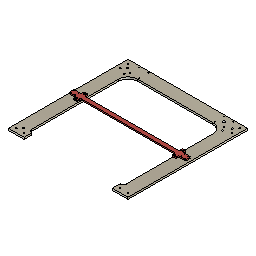
mark 4 top plate nema 23 version (Autodesk Fusion 360 design; units mm, degrees)
Autodesk Fusion 360 part; units mm, degrees
sketch "Sketch1" plane through (0, 0, 0) normal (0, 0, 1) x (1, 0, 0)
  circle A0 centre (2220.6568, 497.0935) radius 8 construction
  circle A1 centre (2186.2292, 516.3803) radius 8 construction
  circle A2 centre (2186.2292, 539.9503) radius 6.25
  line L0 (2209.7992, 516.3803) -> (2162.6592, 516.3803) construction
  circle A3 centre (2209.7992, 516.3803) radius 2.5
  line L1 (2209.7992, 563.5203) -> (2209.7992, 516.3803) construction
  line L2 (2180.9147, 536.6612) -> (2192.6086, 521.2077) construction
  circle A4 centre (2162.6592, 563.5203) radius 2.5
  line L3 (2162.6592, 516.3803) -> (2162.6592, 563.5203) construction
  line L4 (2162.6592, 563.5203) -> (2209.7992, 563.5203) construction
  circle A5 centre (1718.6797, 497.092) radius 8 construction
  circle A6 centre (1753.2073, 516.3788) radius 8 construction
  circle A7 centre (1753.2073, 539.9488) radius 6.25 construction
  line L5 (1729.6373, 516.3788) -> (1776.7773, 563.5188) construction
  line L6 (1729.6373, 516.3788) -> (1776.7773, 516.3788) construction
  circle A8 centre (1729.6373, 516.3788) radius 2.5
  line L7 (1729.6373, 563.5188) -> (1729.6373, 516.3788) construction
  circle A9 centre (1776.7773, 563.5188) radius 2.5
  line L8 (1776.7773, 516.3788) -> (1776.7773, 563.5188) construction
  line L9 (1776.7773, 563.5188) -> (1729.6373, 563.5188) construction
  circle A10 centre (1776.7773, 516.3788) radius 2.5006
  circle A11 centre (1729.6373, 563.5188) radius 2.5006
  circle A12 centre (2209.7992, 563.5203) radius 2.5
  circle A13 centre (2162.6592, 516.3803) radius 2.5
  circle A14 centre (2236.6726, 530.4061) radius 4
  circle A15 centre (1702.7758, 530.4098) radius 4
  circle A16 centre (1718.6797, 497.092) radius 4
  circle A17 centre (2220.6568, 497.0935) radius 4
  circle A18 centre (2236.6726, 530.4061) radius 8 construction
  circle A19 centre (1702.7758, 530.4098) radius 8 construction
  circle A20 centre (2254.5183, 550.8989) radius 3.5
  circle A21 centre (2254.5183, 510.8989) radius 3.5
  circle A22 centre (1685, 550.8955) radius 3.5
  line L10 (1685, 550.8955) -> (1685, 510.8955) construction
  circle A23 centre (1685, 510.8955) radius 3.5
  line L11 (1744.9182, -38.7028) -> (1744.9182, 1.2972)
  line L12 (1744.9182, 1.2972) -> (1743.5, 1.2972)
  line L13 (2194.5182, -38.7028) -> (2194.5182, 1.2972)
  line L14 (2194.5182, 1.2972) -> (2196.0182, 1.2972)
  line L15 (1778.5, 507.7284) -> (2161.0182, 507.7284)
  line L16 (2274.5182, -38.7028) -> (2194.5182, -38.7028)
  line L17 (1744.9182, -38.7028) -> (1664.9182, -38.7028)
  arc A24 (1778.5, 507.7284) -> (1728.5, 457.7284) centre (1778.5, 457.7284) ccw
  arc A25 (2211.0182, 457.7284) -> (2161.0182, 507.7284) centre (2161.0182, 457.7284) ccw
  arc A26 (1728.5, 16.2972) -> (1743.5, 1.2972) centre (1743.5, 16.2972) ccw
  arc A27 (2196.0182, 1.2972) -> (2211.0182, 16.2972) centre (2196.0182, 16.2972) ccw
  circle A28 centre (1684.9182, -18.7028) radius 3.5
  circle A29 centre (1724.9182, -18.7028) radius 3.5
  circle A30 centre (2214.5182, -18.7028) radius 3.5
  circle A31 centre (2254.5182, -18.7028) radius 3.5
  line L18 (2274.5182, -38.7028) -> (2274.5182, 570.8972)
  line L19 (2274.5182, 570.8972) -> (1665, 570.8955)
  line L20 (1665, 570.8955) -> (1664.9182, -38.7028)
  circle A32 centre (2236.6726, 0.4061) radius 8 construction
  line L21 (1672.1777, 267) -> (1672.1777, 284)
  line L22 (2267.1777, 284) -> (2267.1777, 267)
  line L23 (1708.8553, 292) -> (1708.8553, 299)
  line L24 (1712.8553, 303) -> (1724.5, 303)
  line L25 (1728.5, 299) -> (1728.5, 292)
  line L26 (1724.5, 248) -> (1712.8553, 248)
  line L27 (1708.8553, 252) -> (1708.8553, 259)
  line L28 (1728.5, 259) -> (1728.5, 252)
  line L29 (2226.5, 248) -> (2215.0182, 248)
  line L30 (2210.8553, 256.2827) -> (2210.8553, 259)
  line L31 (2210.8553, 263) -> (2211.0182, 263)
  line L32 (2230.5, 259) -> (2230.5, 252)
  line L33 (2210.8553, 248) -> (2211.0182, 248.1244) construction
  line L34 (2211.0182, 288) -> (2210.8553, 288)
  line L35 (2210.8553, 292) -> (2210.8553, 299)
  line L36 (2214.8553, 303) -> (2226.5, 303)
  line L37 (2230.5, 299) -> (2230.5, 292)
  line L38 (2263.1777, 263) -> (2234.5, 263)
  line L39 (2234.5, 288) -> (2263.1777, 288)
  line L40 (2211.0182, 262.8756) -> (2210.8553, 263) construction
  line L41 (1704.8553, 263) -> (1676.1777, 263)
  line L42 (1728.5, 457.7284) -> (1728.5, 292)
  line L43 (1728.5, 259) -> (1728.5, 16.2972)
  line L44 (1676.1777, 288) -> (1704.8553, 288)
  arc A33 (1708.8553, 259) -> (1704.8553, 263) centre (1704.8553, 259) ccw
  arc A34 (1704.8553, 288) -> (1708.8553, 292) centre (1704.8553, 292) ccw
  arc A35 (2230.5, 292) -> (2234.5, 288) centre (2234.5, 292) ccw
  arc A36 (2234.5, 263) -> (2230.5, 259) centre (2234.5, 259) ccw
  arc A37 (2226.5, 248) -> (2230.5, 252) centre (2226.5, 252) ccw
  arc A38 (2211.0182, 252) -> (2215.0182, 248) centre (2215.0182, 252) ccw
  arc A39 (2214.8553, 303) -> (2210.8553, 299) centre (2214.8553, 299) ccw
  arc A40 (2230.5, 299) -> (2226.5, 303) centre (2226.5, 299) ccw
  arc A41 (2263.1777, 263) -> (2267.1777, 267) centre (2263.1777, 267) ccw
  arc A42 (2267.1777, 284) -> (2263.1777, 288) centre (2263.1777, 284) ccw
  arc A43 (1672.1777, 267) -> (1676.1777, 263) centre (1676.1777, 267) ccw
  arc A44 (1676.1777, 288) -> (1672.1777, 284) centre (1676.1777, 284) ccw
  arc A45 (1712.8553, 303) -> (1708.8553, 299) centre (1712.8553, 299) ccw
  arc A46 (1728.5, 299) -> (1724.5, 303) centre (1724.5, 299) ccw
  arc A47 (1724.5, 248) -> (1728.5, 252) centre (1724.5, 252) ccw
  arc A48 (1708.8553, 252) -> (1712.8553, 248) centre (1712.8553, 252) ccw
  line L45 (2211.0182, 262.8756) -> (2211.0182, 263)
  line L46 (2211.0182, 288) -> (2211.0182, 288.1244)
  line L47 (2211.0182, 252) -> (2210.8553, 256.2827)
  circle A49 centre (1718.6777, 295.5) radius 4
  circle A50 centre (1718.6777, 255.5) radius 4
  circle A51 centre (2220.6777, 295.5) radius 4
  circle A52 centre (2220.3553, 255.5) radius 4
  circle A53 centre (2240.6777, 283) radius 1.5
  circle A54 centre (2240.6777, 268) radius 1.5
  circle A55 centre (2260.6777, 268) radius 1.5
  circle A56 centre (2260.6777, 283) radius 1.5
  circle A57 centre (1698.6777, 283) radius 1.5
  circle A58 centre (1698.6777, 268) radius 1.5
  circle A59 centre (1678.6777, 268) radius 1.5
  circle A60 centre (1678.6777, 283) radius 1.5
  circle A61 centre (1718.6777, 255.5) radius 8 construction
  circle A62 centre (1718.6777, 295.5) radius 8 construction
  circle A63 centre (2220.3553, 255.5) radius 8 construction
  circle A64 centre (2220.6777, 295.5) radius 8 construction
  line L48 (2228.3553, 255.5) -> (2228.3553, 0.4062) construction
  line L49 (2244.6726, 0.4059) -> (2244.6726, 530.4061) construction
  line L50 (1664.9159, -55.9986) -> (1702.7616, -56.0037)
  circle A65 centre (1702.7692, 0.4768) radius 4
  circle A66 centre (1702.7692, 0.4768) radius 8 construction
  line L51 (1694.7692, 0.4768) -> (1694.7692, 530.8955) construction
  line L52 (1710.7692, 0.4768) -> (1710.6777, 255.4971) construction
  line L53 (2205.8553, 265.5) -> (1733.5, 265.5)
  line L54 (1733.5, 285.5) -> (2205.8553, 285.5)
  line L55 (1728.5, 292) -> (1728.5, 290.5)
  line L56 (1728.5, 259) -> (1728.5, 260.5)
  line L57 (2210.8553, 292) -> (2210.8553, 290.5)
  line L58 (2210.8553, 259) -> (2210.8553, 260.5)
  arc A67 (1728.5, 290.5) -> (1733.5, 285.5) centre (1733.5, 290.5) ccw
  arc A68 (1733.5, 265.5) -> (1728.5, 260.5) centre (1733.5, 260.5) ccw
  arc A69 (2205.8553, 285.5) -> (2210.8553, 290.5) centre (2205.8553, 290.5) ccw
  arc A70 (2210.8553, 260.5) -> (2205.8553, 265.5) centre (2205.8553, 260.5) ccw
  line L59 (2187.667, 546.0327) -> (2237.888, 538.3132) construction
  line L60 (1710.6777, 295.5) -> (1710.6777, 497.092) construction
  line L61 (2228.6777, 295.5) -> (2228.6777, 497.0935) construction
  line L62 (1748, 523) -> (1758.1512, 536.1251)
  line L63 (1751.7695, 546.0312) -> (1701.5609, 538.317)
  line L64 (1753.2073, 508.3788) -> (2220.6568, 505.0935) construction
  line L65 (2186.2292, 508.3803) -> (1718.6234, 505.0918) construction
  line L66 (1999.6777, 245.5) -> (1939.6777, 245.5) construction
  line L67 (1939.6777, 245.5) -> (1939.6777, 305.5) construction
  line L68 (1939.6777, 305.5) -> (1999.6777, 305.5) construction
  line L69 (1999.6777, 305.5) -> (1999.6777, 245.5) construction
  line L70 (1999.6777, 245.5) -> (1939.6777, 305.5) construction
  line L71 (1939.6777, 245.5) -> (1999.6777, 305.5) construction
  line L72 (2220.6777, 287.5) -> (1999.6777, 287.5) construction
  line L73 (2220.3553, 263.5) -> (1999.6777, 263.5) construction
  line L74 (1718.6777, 263.5) -> (1939.6777, 263.5) construction
  line L75 (1718.6777, 287.5) -> (1939.6777, 287.5) construction
  line L76 (2211.0182, 457.7284) -> (2211.0182, 16.2972)
  line L77 (1728.5, 241.8932) -> (1728.5, 309)
  point P0 (2186.2292, 539.9503)
  point P1 (2220.6568, 505.0935)
  point P2 (2186.2292, 516.3803)
  point P3 (2220.6568, 497.0935)
  point P4 (2186.2292, 516.3803)
  point P5 (2186.2292, 539.9503)
  point P6 (2220.6568, 497.0935)
  point P7 (2186.2292, 539.9503)
  point P8 (2187.667, 546.0327)
  point P9 (2186.2292, 508.3803)
  point P10 (1753.2073, 539.9488)
  point P11 (1722.3963, 504.1763)
  point P12 (1753.2073, 516.3788)
  point P13 (1718.6797, 497.092)
  point P14 (1753.2073, 516.3788)
  point P15 (1753.2073, 539.9488)
  point P16 (1718.6797, 497.092)
  point P17 (1753.2073, 539.9488)
  point P18 (1751.7695, 546.0312)
  point P19 (1753.2073, 508.3788)
  point P20 (2236.6726, 530.4061)
  point P21 (1702.7758, 530.4098)
  point P22 (1724.9182, -18.7028)
  point P23 (1684.9182, -18.7028)
  point P24 (2214.5182, -18.7028)
  point P25 (2254.5182, -18.7028)
  point P26 (1665, 570.8955)
  point P27 (2274.5182, 570.8972)
  point P28 (2236.6726, 0.4061)
  point P29 (1969.6777, 275.5)
  point P30 (1718.6777, 295.5)
  point P31 (1718.6777, 255.5)
  point P32 (2220.6777, 295.5)
  point P33 (2220.3553, 255.5)
  point P34 (1698.6777, 283)
  point P35 (1698.6777, 268)
  point P36 (1678.6777, 283)
  point P37 (1678.6777, 268)
  point P38 (2260.6777, 283)
  point P39 (2260.6777, 268)
  point P40 (2240.6777, 268)
  point P41 (2240.6777, 283)
  point P42 (1672.1777, 288)
  point P43 (2267.1777, 288)
  point P44 (1969.6777, 275.5)
  point P45 (1718.6777, 295.5)
  point P46 (1718.6777, 255.5)
  point P47 (2220.6777, 255.5)
  point P48 (2220.6777, 295.5)
  point P49 (1702.7692, 0.4768)
  point P50 (1969.6777, 275.5)
  point P51 (1969.6777, 275.5)
  dimension "d314" = 47.14
  dimension "d315" = 47.14
  dimension "d316" = 5
  dimension "d317" = 5
  dimension "d318" = 12.5
  dimension "d319" = 16
  dimension "d320" = 16
  dimension "d321" = 47.14
  dimension "d322" = 47.14
  dimension "d323" = 5
  dimension "d324" = 5
  dimension "d325" = 12.5
  dimension "d326" = 16
  dimension "d327" = 16
  dimension "d328" = 5.0013
  dimension "d329" = 5.0013
  dimension "d330" = 5
  dimension "d331" = 5
  dimension "d336" = 8
  dimension "d337" = 8
  dimension "d338" = 8
  dimension "d339" = 8
  dimension "d340" = 16
  dimension "d341" = 16
  dimension "d344" = 7
  dimension "d345" = 40
  dimension "d346" = 7
  dimension "d349" = 7
  dimension "d350" = 40
  dimension "d351" = 7
  dimension "d355" = 80
  dimension "d357" = 80
  dimension "d360" = 50
  dimension "d361" = 50
  dimension "d362" = 15
  dimension "d363" = 15
  dimension "d366" = 40
  dimension "d367" = 7
  dimension "d368" = 7
  dimension "d371" = 40
  dimension "d372" = 7
  dimension "d373" = 7
  dimension "d376" = 530
  dimension "d377" = 16
  dimension "d393" = 502
  dimension "d394" = 40
  dimension "d399" = 20
  dimension "d400" = 20
  dimension "d401" = 595
  dimension "d403" = 8
  dimension "d404" = 8
  dimension "d405" = 8
  dimension "d406" = 8
  dimension "d407" = 3
  dimension "d408" = 3
  dimension "d409" = 3
  dimension "d410" = 3
  dimension "d412" = 3
  dimension "d413" = 3
  dimension "d414" = 3
  dimension "d415" = 3
  dimension "d418" = 16
  dimension "d419" = 16
  dimension "d420" = 16
  dimension "d421" = 16
  dimension "d423" = 37.8457
  dimension "d424" = 8
  dimension "d425" = 16
  dimension "d427" = 5
  dimension "d428" = 5
  dimension "d429" = 5
  dimension "d430" = 5
  dimension "d431" = 60
  dimension "d432" = 60
  constraint horizontal L16
  constraint coincident P7 P5
  constraint perpendicular L0 L3
  constraint parallel L0 L4
  constraint parallel L1 L3
  constraint horizontal L0
  constraint coincident A4.centre L3.end
  constraint coincident L0.start A3.centre
  constraint midpoint P4 L0
  constraint coincident P4 P2
  constraint coincident P6 P3
  constraint coincident P8 A2
  constraint coincident L2.start A2
  constraint coincident L2.end A1
  constraint tangent A1 L2
  constraint coincident P9 A1
  constraint coincident P1 A0
  constraint coincident P17 P15
  constraint perpendicular L6 L8
  constraint parallel L6 L9
  constraint parallel L7 L8
  constraint coincident P17 L5
  constraint coincident L5.end A9.centre
  constraint coincident L5.start L6.start
  constraint midpoint P14 L6
  constraint coincident P14 P12
  constraint coincident P16 P13
  constraint coincident P18 A7
  constraint coincident P19 A6
  constraint coincident P11 A5
  constraint coincident L6.end L8.start
  constraint coincident L7.start L9.end
  constraint coincident L1.start L4.end
  constraint coincident L0.end L3.start
  constraint coincident P20 A14.centre
  constraint coincident P21 A15.centre
  constraint concentric A0 A17
  constraint coincident A22.centre L10.start
  constraint coincident L10.end A23.centre
  constraint perpendicular L16 L42
  constraint vertical L11
  constraint horizontal L12
  constraint vertical L13
  constraint horizontal L14
  constraint collinear L16 L17
  constraint tangent A24 L42
  constraint tangent L15 A24
  constraint tangent L15 A25
  constraint tangent L12 A26
  constraint tangent A26 L42
  constraint tangent L14 A27
  constraint coincident P23 A28.centre
  constraint coincident P22 A29.centre
  constraint coincident P24 A30.centre
  constraint coincident P25 A31.centre
  constraint coincident P27 L18.end
  constraint perpendicular L16 L18
  constraint coincident P26 L19.end
  constraint coincident P28 A32.centre
  constraint coincident A32 L49.start
  constraint perpendicular L21 L38
  constraint parallel L38 L44
  constraint parallel L21 L22
  constraint horizontal L38
  constraint parallel L23 L25
  constraint coincident P45 P30
  constraint perpendicular L26 L27
  constraint parallel L27 L28
  constraint horizontal L26
  constraint perpendicular L29 L30
  constraint parallel L29 L31
  constraint parallel L30 L32
  constraint horizontal L29
  constraint coincident L33 P47
  constraint perpendicular L34 L35
  constraint parallel L34 L36
  constraint parallel L35 L37
  constraint horizontal L34
  constraint coincident P48 P32
  constraint collinear L39 L44
  constraint collinear L42 L43
  constraint tangent L27 A33
  constraint tangent L41 A33
  constraint tangent L44 A34
  constraint tangent L23 A34
  constraint coincident L31.start L30
  constraint coincident L34.end L35
  constraint tangent L37 A35
  constraint tangent L39 A35
  constraint tangent L38 A36
  constraint tangent L32 A36
  constraint tangent L29 A37
  constraint tangent L32 A37
  constraint coincident L33.start L29
  constraint tangent L29 A38
  constraint tangent L35 A39
  constraint tangent L36 A39
  constraint tangent L37 A40
  constraint tangent L36 A40
  constraint tangent L38 A41
  constraint tangent L22 A41
  constraint coincident P43 L22
  constraint coincident P43 L39
  constraint tangent L22 A42
  constraint tangent L39 A42
  constraint tangent L41 A43
  constraint tangent L21 A43
  constraint coincident P42 L21
  constraint coincident P42 L44
  constraint tangent L21 A44
  constraint tangent L44 A44
  constraint tangent L23 A45
  constraint tangent L24 A45
  constraint tangent L25 A46
  constraint tangent L24 A46
  constraint tangent L26 A47
  constraint tangent L28 A47
  constraint tangent L26 A48
  constraint tangent L27 A48
  constraint coincident P46 P31
  constraint coincident P33 A52.centre
  constraint coincident P41 A53.centre
  constraint coincident P40 A54.centre
  constraint coincident P39 A55.centre
  constraint coincident P38 A56.centre
  constraint coincident P34 A57.centre
  constraint coincident P35 A58.centre
  constraint coincident P37 A59.centre
  constraint coincident P36 A60.centre
  constraint concentric A52 A63
  constraint coincident A63 L48.start
  constraint tangent A63 L48
  constraint vertical L48
  constraint coincident A18 L49.end
  constraint tangent A18 L49
  constraint vertical L49
  constraint perpendicular L20 L50
  constraint coincident P49 A65.centre
  constraint concentric A65 A66
  constraint coincident A66 L51.start
  constraint tangent A66 L51
  constraint parallel L10 L51
  constraint coincident A66 L52.start
  constraint coincident A61 L52.end
  constraint tangent A61 L52
  constraint parallel L53 L54
  constraint horizontal L53
  constraint coincident P51 P50
  constraint perpendicular L54 L55
  constraint perpendicular L53 L56
  constraint perpendicular L54 L57
  constraint perpendicular L53 L58
  constraint tangent L54 A67
  constraint tangent L55 A67
  constraint tangent L53 A68
  constraint tangent L56 A68
  constraint tangent L54 A69
  constraint tangent L57 A69
  constraint tangent L53 A70
  constraint tangent L58 A70
  constraint coincident P8 L59.start
  constraint coincident A18 L59.end
  constraint tangent A18 L59
  constraint coincident A62 L60.start
  constraint tangent A62 L60
  constraint vertical L60
  constraint coincident A64 L61.start
  constraint tangent A64 L61
  constraint vertical L61
  constraint coincident A7 L62.end
  constraint tangent A7 L62
  constraint coincident P18 L63.start
  constraint coincident A19 L63.end
  constraint tangent A19 L63
  constraint coincident P19 L64.start
  constraint coincident P1 L64.end
  constraint coincident P9 L65.start
  constraint coincident A5 L65.end
  constraint tangent A5 L65
  constraint perpendicular L66 L67
  constraint parallel L66 L68
  constraint parallel L67 L69
  constraint horizontal L66
  constraint coincident L70 P51
  constraint coincident L71 P51
  constraint coincident A64 L72.start
  constraint coincident L69 L72.end
  constraint tangent A64 L72
  constraint perpendicular L69 L72
  constraint coincident A63 L73.start
  constraint coincident L69 L73.end
  constraint tangent A63 L73
  constraint perpendicular L69 L73
  constraint coincident A61 L74.start
  constraint coincident L67 L74.end
  constraint tangent A61 L74
  constraint perpendicular L67 L74
  constraint coincident A62 L75.start
  constraint coincident L67 L75.end
  constraint tangent A62 L75
  constraint perpendicular L67 L75
  constraint tangent A27 L76
  constraint coincident L43 L77.start
  constraint coincident L42 L77.end
  measures "d314" distance of A4.centre L0.end
  measures "d315" distance of A4.centre L1.start
  measures "d316" diameter of A4
  measures "d317" diameter of A3
  measures "d318" diameter of A2
  measures "d319" diameter of A1
  measures "d320" diameter of A0
  measures "d321" distance of L5.end L6.end
  measures "d322" distance of L5.end L7.start
  measures "d323" diameter of A9
  measures "d324" diameter of A8
  measures "d325" diameter of A7
  measures "d326" diameter of A6
  measures "d327" diameter of A5
  measures "d328" diameter of A10
  measures "d329" diameter of A11
  measures "d330" diameter of A12
  measures "d331" diameter of A13
  measures "d336" diameter of A14
  measures "d337" diameter of A15
  measures "d338" diameter of A16
  measures "d339" diameter of A17
  measures "d340" diameter of A18
  measures "d341" diameter of A19
  measures "d344" diameter of A20
  measures "d345" distance of A20.centre A21.centre
  measures "d346" diameter of A21
  measures "d349" diameter of A22
  measures "d350" distance of A22.centre L10.end
  measures "d351" diameter of A23
  measures "d355" distance of L17.end L11.start
  measures "d357" distance of L16.start L13.start
  measures "d360" radius of A24
  measures "d361" radius of A25
  measures "d362" radius of A26
  measures "d363" radius of A27
  measures "d366" distance of P22 P23
  measures "d367" diameter of A28
  measures "d368" diameter of A29
  measures "d371" distance of P24 P25
  measures "d372" diameter of A30
  measures "d373" diameter of A31
  measures "d376" distance of P20 P28
  measures "d377" diameter of A32
  measures "d393" distance of P45 P48
  measures "d394" distance of P45 P46
  measures "d399" distance of P38 P41
  measures "d400" distance of P34 P36
  measures "d401" distance of P42 P43
  measures "d403" diameter of A49
  measures "d404" diameter of A50
  measures "d405" diameter of A51
  measures "d406" diameter of A52
  measures "d407" diameter of A53
  measures "d408" diameter of A54
  measures "d409" diameter of A55
  measures "d410" diameter of A56
  measures "d412" diameter of A57
  measures "d413" diameter of A58
  measures "d414" diameter of A59
  measures "d415" diameter of A60
  measures "d418" diameter of A61
  measures "d419" diameter of A62
  measures "d420" diameter of A63
  measures "d421" diameter of A64
  measures "d423" distance of L50.start L50.end
  measures "d424" diameter of A65
  measures "d425" diameter of A66
  measures "d427" radius of A67
  measures "d428" radius of A68
  measures "d429" radius of A69
  measures "d430" radius of A70
  measures "d431" distance of L67.end L68.end
  measures "d432" distance of L66.end L67.end
extrude "Extrude6" add sketch "Sketch1" along normal blind 9.52 contours L11 L12 L13 L14 L15 L16 L17 A24 A25 A26 A27 L18 L19 L20 L21 L22 L23 L24 L26 L27 L29 L32 L36 L37 L38 L39 L41 L42 L43 L44 A33 A34 A35 A36 A37 A38 A39 A40 A41 A42 A43 A44 A45 A46 A47 A48 L76 L77 | L21 L23 L24 L25 L26 L27 L28 L41 L42 L43 L44 A33 A34 A43 A44 A45 A46 A47 A48 L55 L56 L77 | L22 L29 L32 L36 L37 L38 L39 A35 A36 A37 A38 A39 A40 A41 A42 L45 L46 L76 | A49 | A50 | A51 | A52 | A53 | A54 | A55 | A56 | A57 | A58 | A59 | A60 makes body 1
sketch "Sketch10" plane through (0, 0, 0) normal (0, 0, 1) x (1, 0, 0)
sketch "Sketch11" plane through (0, 0, 0) normal (0, 0, 1) x (1, 0, 0)
sketch "Sketch12" plane through (0, 0, 0) normal (0, 0, 1) x (1, 0, 0)
sketch "Sketch13" plane through (0, 0, 0) normal (0, 0, 1) x (1, 0, 0)
sketch "Sketch14" plane through (0, 0, 0) normal (0, 0, 1) x (1, 0, 0)
sketch "Sketch15" plane through (0, 0, 0) normal (0, 0, 1) x (1, 0, 0)
extrude "Extrude4" add sketch "Sketch1" along normal blind 6.35 separate body contours L21 L23 L24 L25 L26 L27 L28 L41 L42 L43 L44 A33 A34 A43 A44 A45 A46 A47 A48 L55 L56 L77 | L30 L35 A39 L45 L46 L47 L53 L54 L57 L58 A67 A68 A69 A70 L76 L77 makes body 2
move_body "Move1" bodies 1 to x (1, 0, 0) y (0, 1, 0) z (0, 0, 1) at (0, 0, -15)
extrude "Extrude7" add sketch "Sketch1" along normal blind 6.35 contours L22 L29 L32 L36 L37 L38 L39 A35 A36 A37 A38 A39 A40 A41 A42 L45 L46 L76 bodies 2
